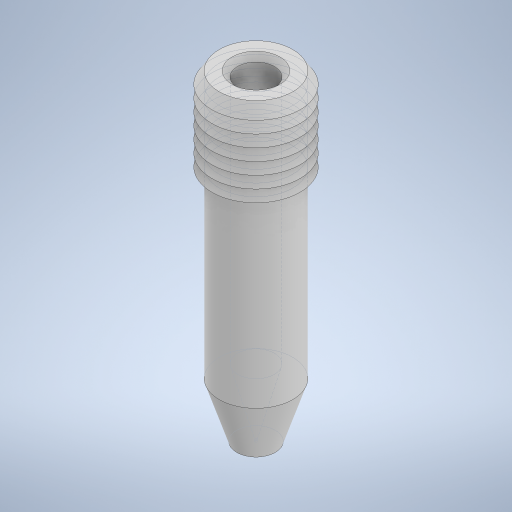
# Autodesk Inventor part: nozzle_with_hose_barb
Saved by Autodesk Inventor 2024.2 (Build 282272000, 272)
## iProperties
Created: 2024-04-22
Part Number: nozzle_with_hose_barb
Material: Generic
Document SubType Name: Modeling
Designer: vasily
Density: 1 g/cm^3
Appearance: Default
Author: vasily
Autodesk Inventor part; units mm, degrees
ref_plane "YZ Plane" through (0, 0, 0) normal (1, 0, 0) x (0, 1, 0)
ref_plane "XZ Plane" through (0, 0, 0) normal (0, 1, 0) x (-1, 0, 0)
ref_plane "XY Plane" through (0, 0, 0) normal (0, 0, 1) x (1, 0, 0)
sketch "Sketch1" plane through (0, 0, 0) normal (0, 0, 1) x (1, 0, 0)
  line L0 (4, 5.9492) -> (4, 35.0492)
  line L1 (0, 0) -> (0, 32.7561)
  line L2 (4, 35.0492) -> (0, 35.0492) construction
  line L3 (4, 35.0492) -> (2.6, 35.0492)
  line L4 (2, 34.4492) -> (2, 7.3356)
  line L5 (2, 7.3356) -> (0.1, 0.2061)
  line L6 (0.1, 0.2061) -> (0.1, 0)
  line L7 (4, 35.0492) -> (4.8, 33.7492)
  line L8 (4.8, 33.7492) -> (4, 33.7492)
  line L9 (4, 33.7492) -> (4.8, 32.4492)
  line L10 (4.8, 32.4492) -> (4, 32.4492)
  line L11 (4, 32.4492) -> (4.8, 31.1492)
  line L12 (4.8, 31.1492) -> (4, 31.1492)
  line L13 (4, 31.1492) -> (4.8, 29.8492)
  line L14 (4.8, 29.8492) -> (4, 29.8492)
  line L15 (4, 29.8492) -> (4.8, 28.5492)
  line L16 (4.8, 28.5492) -> (4, 28.5492)
  line L17 (0, 0) -> (22.3687, 0) construction
  line L18 (0.1, 0) -> (2.1, 0)
  line L19 (2.1, 0) -> (4, 5.9492)
  line L20 (2, 34.4492) -> (2.6, 35.0492)
  line L21 (4.8, 27.2492) -> (4, 27.2492)
  line L22 (4, 28.5492) -> (4.8, 27.2492)
  line L23 (4.8, 25.9492) -> (4, 25.9492)
  line L24 (4, 27.2492) -> (4.8, 25.9492)
  point P0 (2, 35.0492)
  point P1 (22.3687, -1.3)
  point P2 (22.3687, -2.6)
  dimension "d3" = 0.2
  dimension "d4" = 2
  dimension "d7" = 1.3
  dimension "d12" = 1.3
  dimension "d13" = 0
  dimension "d14" = 0.8
  dimension "d17" = 8
  dimension "d19" = 0.6
  dimension "d20" = 0.6
  dimension "d24" = 1.3
  dimension "d29" = 20
  dimension "d30" = 2
  constraints: 50 end point, 9 point on line, 6 vertical, 2 perpendicular, 1 horizontal, 1 midpoint, 32 other
  measures "d3" diameter of L6.end L1
  measures "d4" distance between parallel lines of L4 L0
  measures "d7" distance of L7.end L9.end
  measures "d12" vertical distance of L0.end L7.end
  measures "d13" vertical distance of L7.end L8.end
  measures "d14" horizontal distance of L0.end L7.end
  measures "d17" diameter of L0 L1
  measures "d19" distance of L4.start point (2, 35.049)
  measures "d20" distance of L3.end point (2, 35.049)
  measures "d24" distance of L15.end L21.start
  measures "d29" distance of L23.end L0.start
  measures "d30" distance of L6.end L18.end
revolve "Revolution1" add sketch "Sketch1" angle 360 about axis through (0, 0, 0) along (0, 1, 0)
equation "\"d7\" = d12"
equation "\"d20\" = d19"
equation "\"d24\" = d7"
body "Solid1"
